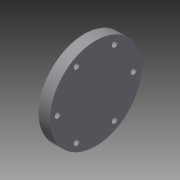
# Autodesk Inventor part: fork
Saved by Autodesk Inventor 2013 (Build 170138000, 138)
## iProperties
Created: 2013-01-09
Part Number: fork
Material: Generic
Document SubType Name: Modeling
Designer: Nano
Density: 1 g/cm^3
Author: Nano
Autodesk Inventor part; units mm, degrees
ref_plane "YZ Plane" through (0, 0, 0) normal (1, 0, 0) x (0, 1, 0)
ref_plane "XZ Plane" through (0, 0, 0) normal (0, 1, 0) x (-1, 0, 0)
ref_plane "XY Plane" through (0, 0, 0) normal (0, 0, 1) x (1, 0, 0)
sketch "Sketch1" plane through (0, 0, 0) normal (1, 0, 0) x (0, 1, 0)
  circle A0 centre (-479.4213, -671.0964) radius 25.4
  circle A1 centre (-479.4213, -671.0964) radius 88.9 projected
  circle A2 centre (-479.4213, -649.9452) radius 1.5875
  circle A3 centre (-497.7388, -660.5208) radius 1.5875
  circle A4 centre (-497.7388, -681.6721) radius 1.5875
  circle A5 centre (-479.4213, -692.2477) radius 1.5875
  circle A6 centre (-461.1038, -681.6721) radius 1.5875
  circle A7 centre (-461.1038, -660.5208) radius 1.5875
  point P0 (0, 0)
  dimension "d0" = 50.8
  dimension "d1" = 3.175
  dimension "d4" = 360
  constraints: 7 centre point, 1 concentric, 13 other
  measures "d0" diameter of A0
  measures "d1" diameter of A2
extrude "Extrusion1" add sketch "Sketch1" along normal blind 6.35 contours A0
sketch "Sketch2" plane through (6.35, -479.4213, -671.0964) normal (1, 0, 0) x (0, 0, -1)
  circle A0 centre (-21.1512, 0) radius 1.5875 projected
  spline S0 degree 3 poles (-5.6187, -9.891) (-73.0206, -34.6538) (-119.0516, 78.5765) (-145.3355, 88.8855) knots 0 0 0 0 1 1 1 1
  spline S1 degree 3 poles (0, 11.5539) (-60.9983, -36.2975) (-102.9311, 114.869) (-133.6383, 103.832) knots 0 0 0 0 1 1 1 1
  line L0 (-145.3355, 88.8855) -> (-133.6383, 103.832)
  arc A1 (-5.6187, -9.891) -> (0, 11.5539) centre (0.2097, 0.0404) ccw
  point P0 (-671.0964, 479.4213)
  point P1 (-69.3034, 5.0557)
  point P2 (-121.2912, 64.8414)
  point P3 (-55.007, 16.7301)
  point P4 (-109.594, 88.8855)
  constraints: 2 end point, 2 point on circle, 1 centre point, 8 other
extrude "Extrusion2" add sketch "Sketch2" along normal blind 19.05
body "Solid1"
